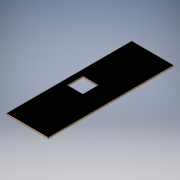
# Autodesk Inventor part: backBoard
Saved by Autodesk Inventor 2016 (Build 200138000, 138)
## iProperties
Created: 2016-12-21
Part Number: backBoard
Material: Wood (Birch)
Document SubType Name: Modeling
Designer: Naga
Density: 0.55 g/cm^3
Appearance: Birch - Natural Polished
Author: Naga
Autodesk Inventor part; units mm, degrees
ref_plane "YZ Plane" through (0, 0, 0) normal (1, 0, 0) x (0, 1, 0)
ref_plane "XZ Plane" through (0, 0, 0) normal (0, 1, 0) x (-1, 0, 0)
ref_plane "XY Plane" through (0, 0, 0) normal (0, 0, 1) x (1, 0, 0)
sketch "Sketch1" plane through (0, 0, 0) normal (0, 1, 0) x (-1, 0, 0)
  line L0 (0, 0) -> (406.4, 0)
  line L1 (406.4, 0) -> (406.4, -1219.2)
  line L2 (406.4, -1219.2) -> (0, -1219.2)
  line L3 (0, -1219.2) -> (0, 0)
  line L4 (0, -609.6) -> (101.6, -609.6)
  line L5 (101.6, -609.6) -> (184.15, -609.6)
  line L6 (184.15, -609.6) -> (273.05, -609.6)
  line L7 (349.25, -533.4) -> (196.85, -533.4)
  line L8 (196.85, -533.4) -> (196.85, -685.8)
  line L9 (196.85, -685.8) -> (349.25, -685.8)
  line L10 (349.25, -685.8) -> (349.25, -533.4)
  line L11 (349.25, -533.4) -> (196.85, -685.8) construction
  line L12 (196.85, -533.4) -> (349.25, -685.8) construction
  dimension "d0" = 1219.2
  dimension "d1" = 406.4
  dimension "d2" = 101.6
  dimension "d3" = 82.55
  dimension "d4" = 88.9
  dimension "d5" = 152.4
  dimension "d6" = 152.4
  constraints: 26 end point, 5 horizontal, 4 parallel, 3 midpoint, 2 perpendicular
  measures "d0" distance of L0.end L1.end
  measures "d1" distance of L1.end L2.end
  measures "d2" distance of L4.start L4.end
  measures "d3" distance of L4.end L5.end
  measures "d4" distance of L5.end L6.end
  measures "d5" distance of L9.end L8.end
  measures "d6" distance of L8.end L7.end
extrude "Extrusion1" add sketch "Sketch1" along normal blind 12.7
body "Solid1"
